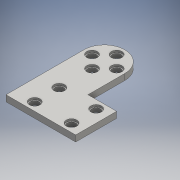
# Autodesk Inventor part: Wheel_holder
Saved by Autodesk Inventor 2016 (Build 200138000, 138)
## iProperties
Created: 2016-05-04
Part Number: Wheel_holder
Material: Generic
Document SubType Name: Modeling
Designer: sunilr
Density: 1 g/cm^3
Appearance: Default
Author: sunilr
Autodesk Inventor part; units mm, degrees
note: some values were not read from the file. Chosen so that the rebuilt part matches the saved one: sketch regions of "Extrusion1".
ref_plane "YZ Plane" through (0, 0, 0) normal (1, 0, 0) x (0, 1, 0)
ref_plane "XZ Plane" through (0, 0, 0) normal (0, 1, 0) x (-1, 0, 0)
ref_plane "XY Plane" through (0, 0, 0) normal (0, 0, 1) x (1, 0, 0)
sketch "Sketch1" plane through (0, 0, 0) normal (0, 0, 1) x (1, 0, 0)
  circle A0 centre (0, 0) radius 10
  line L0 (10, 0) -> (10, -38)
  line L1 (10, -38) -> (-10, -38)
  line L2 (-10, -38) -> (-10, 0)
  circle A1 centre (0, 6) radius 2.1
  circle A2 centre (-6, 0) radius 2.1
  circle A3 centre (6, 0) radius 2.1
  circle A4 centre (0, -6) radius 2.1
  circle A5 centre (0, -22) radius 2.1
  circle A6 centre (0, -34) radius 2.1
  line L3 (10, -18) -> (24, -18)
  line L4 (24, -18) -> (24, -38)
  line L5 (24, -38) -> (10, -38)
  line L6 (10, -38) -> (10, -18)
  circle A7 centre (18, -22) radius 2.1
  circle A8 centre (18, -34) radius 2.1
  line L7 (-10, 0) -> (-8.1, 0)
  line L8 (-3.9, 0) -> (3.9, 0)
  line L9 (8.1, 0) -> (10, 0)
  dimension "d0" = 20
  dimension "d1" = 38
  dimension "d2" = 4.2
  dimension "d3" = 4.2
  dimension "d4" = 4.2
  dimension "d5" = 4.2
  dimension "d6" = 4.2
  dimension "d7" = 4.2
  dimension "d8" = 14
  dimension "d9" = 4.2
  dimension "d10" = 4.2
  constraints: 20 end point, 8 centre point, 6 parallel, 4 horizontal, 4 perpendicular, 4 point on circle, 1 coincident, 1 horizontal alignment, 2 other
  measures "d1" distance of L0.start L0.end
  measures "d2" diameter of A1
  measures "d3" diameter of A2
  measures "d4" diameter of A3
  measures "d5" diameter of A4
  measures "d6" diameter of A5
  measures "d7" diameter of A6
  measures "d8" distance of L4.end L5.end
  measures "d9" diameter of A7
  measures "d10" diameter of A8
extrude "Extrusion1" add sketch "Sketch1" along normal blind 3 contours L9 A3 L8 A2 L7 A0 | L0 L1 L2 A0 | A0 L7 A2 L8 A3 L9 | L3 L4 L5 L0
sketch "Sketch2" plane through (0, 0, 3) normal (0, 0, 1) x (1, 0, 0)
  circle A0 centre (0, 6) radius 2.6
  circle A1 centre (-6, 0) radius 2.6
  circle A2 centre (6, 0) radius 2.6
  circle A3 centre (0, -6) radius 2.6
  circle A4 centre (0, -22) radius 2.6
  circle A5 centre (0, -34) radius 2.6
  circle A6 centre (18, -22) radius 2.6
  circle A7 centre (18, -34) radius 2.6
  point P0 (0, 0)
  dimension "d13" = 5.2
  dimension "d14" = 5.2
  dimension "d15" = 5.2
  dimension "d16" = 5.2
  dimension "d17" = 5.2
  dimension "d18" = 5.2
  dimension "d19" = 5.2
  dimension "d20" = 5.2
  constraints: 8 centre point
  measures "d13" diameter of A0
  measures "d14" diameter of A1
  measures "d15" diameter of A2
  measures "d16" diameter of A3
  measures "d17" diameter of A4
  measures "d18" diameter of A5
  measures "d19" diameter of A6
  measures "d20" diameter of A7
extrude "Extrusion2" cut sketch "Sketch2" against normal blind 1
body "Solid1"
